Autodesk Inventor part; units mm, degrees
(part 3 of 5)
sketch "Sketch8" plane through (0, 0, 3) normal (0, 0, 1) x (1, 0, 0)
  line L0 (80.4, 215) -> (-78, 215) projected
  line L1 (-78, 215) -> (-78, 46.0635) projected
  line L2 (-78, 46.0635) -> (-75, 46.0635) projected
  line L3 (-75, 46.0635) -> (-75, 40.8932) projected
  line L4 (-75, 40.8932) -> (-78, 40.8932) projected
  line L5 (-78, 40.8932) -> (-78, 30.6062) projected
  line L6 (-78, 30.6062) -> (-75, 30.6062) projected
  line L7 (-75, 30.6062) -> (-75, 20.5478) projected
  line L8 (-75, 20.5478) -> (-78, 20.5478) projected
  line L9 (-78, 20.5478) -> (-78, 10.2608) projected
  line L10 (-78, 10.2608) -> (-75, 10.2608) projected
  line L11 (-75, 10.2608) -> (-75, -0.1068) projected
  line L12 (-75, -0.1068) -> (-78, -0.1068) projected
  line L13 (-78, -0.1068) -> (-78, -10.3938) projected
  line L14 (-78, -10.3938) -> (-75, -10.3938) projected
  line L15 (-75, -10.3938) -> (-75, -20.4522) projected
  line L16 (-75, -20.4522) -> (-78, -20.4522) projected
  line L17 (-78, -20.4522) -> (-78, -30.7392) projected
  line L18 (-78, -30.7392) -> (-75, -30.7392) projected
  line L19 (-75, -30.7392) -> (-75, -41.1068) projected
  line L20 (-75, -41.1068) -> (-78, -41.1068) projected
  line L21 (-78, -41.1068) -> (-78, -51.3938) projected
  line L22 (-78, -51.3938) -> (-75, -51.3938) projected
  line L23 (-75, -51.3938) -> (-75, -61.4522) projected
  line L24 (-75, -61.4522) -> (-78, -61.4522) projected
  line L25 (-78, -61.4522) -> (-78, -71.7392) projected
  line L26 (-78, -71.7392) -> (-75, -71.7392) projected
  line L27 (-75, -71.7392) -> (-75, -82.1068) projected
  line L28 (-75, -82.1068) -> (-78, -82.1068) projected
  line L29 (-78, -82.1068) -> (-78, -92.3938) projected
  line L30 (-78, -92.3938) -> (-75, -92.3938) projected
  line L31 (-75, -92.3938) -> (-75, -102.4522) projected
  line L32 (-75, -102.4522) -> (-78, -102.4522) projected
  line L33 (-78, -102.4522) -> (-78, -112.7392) projected
  line L34 (-78, -112.7392) -> (-75, -112.7392) projected
  line L35 (-75, -112.7392) -> (-75, -130) projected
  line L36 (-75, -130) -> (-25.3933, -130) projected
  line L37 (-25.3933, -130) -> (-25.3933, -147.5) projected
  line L38 (-25.3933, -147.5) -> (23.6067, -147.5) projected
  line L39 (23.6067, -147.5) -> (23.6067, -130) projected
  line L40 (23.6067, -130) -> (98, -130) projected
  line L41 (98, -130) -> (98, 184.5) projected
  line L42 (98, 184.5) -> (80.4, 184.5) projected
  line L43 (80.4, 184.5) -> (80.4, 215) projected
  circle A0 centre (88, 174.5) radius 2.25 projected
  circle A1 centre (88, 131.8987) radius 2.25 projected
  circle A2 centre (88, 58.3987) radius 2.25 projected
  circle A3 centre (88, -117.6237) radius 2.25 projected
  circle A4 centre (-19.3694, 126.1487) radius 1.2 projected
  circle A5 centre (52.1306, 126.1487) radius 1.2 projected
  circle A6 centre (52.1306, 137.6487) radius 1.2 projected
  circle A7 centre (52.1306, 209.1487) radius 1.2 projected
  circle A8 centre (52.1306, 54.6487) radius 1.2 projected
  circle A9 centre (-19.3694, 137.6487) radius 1.2 projected
  circle A10 centre (-19.3694, 209.1487) radius 1.2 projected
  circle A11 centre (-19.3694, 54.6487) radius 1.2 projected
  circle A12 centre (-17.8933, -140) radius 2.25 projected
  circle A13 centre (16.1067, -140) radius 2.25 projected
  line L44 (-58.9404, 10.4643) -> (-58.9404, 20.3443) projected
  arc A14 (-55.9404, 23.3443) -> (-58.9404, 20.3443) centre (-55.9404, 20.3443) ccw projected
  line L45 (-55.9404, 23.3443) -> (31.7396, 23.3443) projected
  arc A15 (34.7396, 20.3443) -> (31.7396, 23.3443) centre (31.7396, 20.3443) ccw projected
  line L46 (34.7396, 20.3443) -> (34.7396, 10.4643) projected
  arc A16 (31.7396, 7.4643) -> (34.7396, 10.4643) centre (31.7396, 10.4643) ccw projected
  line L47 (31.7396, 7.4643) -> (-55.9404, 7.4643) projected
  arc A17 (-58.9404, 10.4643) -> (-55.9404, 7.4643) centre (-55.9404, 10.4643) ccw projected
  line L48 (-58.9404, 30.8097) -> (-58.9404, 40.6897) projected
  arc A18 (-55.9404, 43.6897) -> (-58.9404, 40.6897) centre (-55.9404, 40.6897) ccw projected
  line L49 (-55.9404, 43.6897) -> (31.7396, 43.6897) projected
  arc A19 (34.7396, 40.6897) -> (31.7396, 43.6897) centre (31.7396, 40.6897) ccw projected
  line L50 (34.7396, 40.6897) -> (34.7396, 30.8097) projected
  arc A20 (31.7396, 27.8097) -> (34.7396, 30.8097) centre (31.7396, 30.8097) ccw projected
  line L51 (31.7396, 27.8097) -> (-55.9404, 27.8097) projected
  arc A21 (-58.9404, 30.8097) -> (-55.9404, 27.8097) centre (-55.9404, 30.8097) ccw projected
  arc A22 (-55.9404, 2.9989) -> (-58.9404, -0.0011) centre (-55.9404, -0.0011) ccw projected
  line L52 (-55.9404, 2.9989) -> (31.7396, 2.9989) projected
  arc A23 (34.7396, -0.0011) -> (31.7396, 2.9989) centre (31.7396, -0.0011) ccw projected
  line L53 (34.7396, -0.0011) -> (34.7396, -9.8811) projected
  arc A24 (31.7396, -12.8811) -> (34.7396, -9.8811) centre (31.7396, -9.8811) ccw projected
  line L54 (31.7396, -12.8811) -> (-55.9404, -12.8811) projected
  arc A25 (-58.9404, -9.8811) -> (-55.9404, -12.8811) centre (-55.9404, -9.8811) ccw projected
  line L55 (-58.9404, -9.8811) -> (-58.9404, -0.0011) projected
  arc A26 (-55.9404, -37.6919) -> (-58.9404, -40.6919) centre (-55.9404, -40.6919) ccw projected
  line L56 (-55.9404, -37.6919) -> (31.7396, -37.6919) projected
  arc A27 (34.7396, -40.6919) -> (31.7396, -37.6919) centre (31.7396, -40.6919) ccw projected
  line L57 (34.7396, -40.6919) -> (34.7396, -50.5719) projected
  arc A28 (31.7396, -53.5719) -> (34.7396, -50.5719) centre (31.7396, -50.5719) ccw projected
  line L58 (31.7396, -53.5719) -> (-55.9404, -53.5719) projected
  arc A29 (-58.9404, -50.5719) -> (-55.9404, -53.5719) centre (-55.9404, -50.5719) ccw projected
  line L59 (-58.9404, -50.5719) -> (-58.9404, -40.6919) projected
  line L60 (-55.9404, -58.0373) -> (31.7396, -58.0373) projected
  arc A30 (34.7396, -61.0373) -> (31.7396, -58.0373) centre (31.7396, -61.0373) ccw projected
  line L61 (34.7396, -61.0373) -> (34.7396, -70.9173) projected
  arc A31 (31.7396, -73.9173) -> (34.7396, -70.9173) centre (31.7396, -70.9173) ccw projected
  line L62 (31.7396, -73.9173) -> (-55.9404, -73.9173) projected
  arc A32 (-58.9404, -70.9173) -> (-55.9404, -73.9173) centre (-55.9404, -70.9173) ccw projected
  line L63 (-58.9404, -70.9173) -> (-58.9404, -61.0373) projected
  arc A33 (-55.9404, -58.0373) -> (-58.9404, -61.0373) centre (-55.9404, -61.0373) ccw projected
  line L64 (31.7396, -33.2265) -> (-55.9404, -33.2265) projected
  arc A34 (-58.9404, -30.2265) -> (-55.9404, -33.2265) centre (-55.9404, -30.2265) ccw projected
  line L65 (-58.9404, -30.2265) -> (-58.9404, -20.3465) projected
  arc A35 (-55.9404, -17.3465) -> (-58.9404, -20.3465) centre (-55.9404, -20.3465) ccw projected
  line L66 (-55.9404, -17.3465) -> (31.7396, -17.3465) projected
  arc A36 (34.7396, -20.3465) -> (31.7396, -17.3465) centre (31.7396, -20.3465) ccw projected
  line L67 (34.7396, -20.3465) -> (34.7396, -30.2265) projected
  arc A37 (31.7396, -33.2265) -> (34.7396, -30.2265) centre (31.7396, -30.2265) ccw projected
  arc A38 (34.7396, -81.3827) -> (31.7396, -78.3827) centre (31.7396, -81.3827) ccw projected
  line L68 (34.7396, -81.3827) -> (34.7396, -91.2627) projected
  arc A39 (31.7396, -94.2627) -> (34.7396, -91.2627) centre (31.7396, -91.2627) ccw projected
  line L69 (31.7396, -94.2627) -> (-55.9404, -94.2627) projected
  arc A40 (-58.9404, -91.2627) -> (-55.9404, -94.2627) centre (-55.9404, -91.2627) ccw projected
  line L70 (-58.9404, -91.2627) -> (-58.9404, -81.3827) projected
  arc A41 (-55.9404, -78.3827) -> (-58.9404, -81.3827) centre (-55.9404, -81.3827) ccw projected
  line L71 (-55.9404, -78.3827) -> (31.7396, -78.3827) projected
  arc A42 (31.7396, -114.6081) -> (34.7396, -111.6081) centre (31.7396, -111.6081) ccw projected
  line L72 (31.7396, -114.6081) -> (-55.9404, -114.6081) projected
  arc A43 (-58.9404, -111.6081) -> (-55.9404, -114.6081) centre (-55.9404, -111.6081) ccw projected
  line L73 (-58.9404, -111.6081) -> (-58.9404, -101.7281) projected
  arc A44 (-55.9404, -98.7281) -> (-58.9404, -101.7281) centre (-55.9404, -101.7281) ccw projected
  line L74 (-55.9404, -98.7281) -> (31.7396, -98.7281) projected
  arc A45 (34.7396, -101.7281) -> (31.7396, -98.7281) centre (31.7396, -101.7281) ccw projected
  line L75 (34.7396, -101.7281) -> (34.7396, -111.6081) projected
  arc A46 (-6.9692, 54.8876) -> (4.019, 51.5987) centre (4.019, 71.5987) ccw projected
  arc A47 (-13.8416, 60.5179) -> (-6.9692, 54.8876) centre (16.3806, 90.3987) ccw projected
  arc A48 (-19.6194, 74.5794) -> (-13.8416, 60.5179) centre (0.3806, 74.5794) ccw projected
  line L76 (-19.6194, 74.5794) -> (-19.6194, 106.218) projected
  arc A49 (-13.8416, 120.2796) -> (-19.6194, 106.218) centre (0.3806, 106.218) ccw projected
  arc A50 (-6.9692, 125.9099) -> (-13.8416, 120.2796) centre (16.3806, 90.3987) ccw projected
  arc A51 (4.019, 129.1987) -> (-6.9692, 125.9099) centre (4.019, 109.1987) ccw projected
  line L77 (4.019, 129.1987) -> (28.7422, 129.1987) projected
  arc A52 (39.7304, 125.9099) -> (28.7422, 129.1987) centre (28.7422, 109.1987) ccw projected
  arc A53 (46.6028, 120.2796) -> (39.7304, 125.9099) centre (16.3806, 90.3987) ccw projected
  arc A54 (52.3806, 106.218) -> (46.6028, 120.2796) centre (32.3806, 106.218) ccw projected
  line L78 (52.3806, 106.218) -> (52.3806, 74.5794) projected
  arc A55 (46.6028, 60.5179) -> (52.3806, 74.5794) centre (32.3806, 74.5794) ccw projected
  arc A56 (39.7304, 54.8876) -> (46.6028, 60.5179) centre (16.3806, 90.3987) ccw projected
  arc A57 (28.7422, 51.5987) -> (39.7304, 54.8876) centre (28.7422, 71.5987) ccw projected
  line L79 (28.7422, 51.5987) -> (4.019, 51.5987) projected
  arc A58 (-6.9692, 137.8876) -> (4.019, 134.5987) centre (4.019, 154.5987) ccw projected
  arc A59 (-13.8416, 143.5179) -> (-6.9692, 137.8876) centre (16.3806, 173.3987) ccw projected
  arc A60 (-19.6194, 157.5794) -> (-13.8416, 143.5179) centre (0.3806, 157.5794) ccw projected
  line L80 (-19.6194, 157.5794) -> (-19.6194, 189.218) projected
  arc A61 (-13.8416, 203.2796) -> (-19.6194, 189.218) centre (0.3806, 189.218) ccw projected
  arc A62 (-6.9692, 208.9099) -> (-13.8416, 203.2796) centre (16.3806, 173.3987) ccw projected
  arc A63 (4.019, 212.1987) -> (-6.9692, 208.9099) centre (4.019, 192.1987) ccw projected
  line L81 (4.019, 212.1987) -> (28.7422, 212.1987) projected
  arc A64 (39.7304, 208.9099) -> (28.7422, 212.1987) centre (28.7422, 192.1987) ccw projected
  arc A65 (46.6028, 203.2796) -> (39.7304, 208.9099) centre (16.3806, 173.3987) ccw projected
  arc A66 (52.3806, 189.218) -> (46.6028, 203.2796) centre (32.3806, 189.218) ccw projected
  line L82 (52.3806, 189.218) -> (52.3806, 157.5794) projected
  arc A67 (46.6028, 143.5179) -> (52.3806, 157.5794) centre (32.3806, 157.5794) ccw projected
  arc A68 (39.7304, 137.8876) -> (46.6028, 143.5179) centre (16.3806, 173.3987) ccw projected
  arc A69 (28.7422, 134.5987) -> (39.7304, 137.8876) centre (28.7422, 154.5987) ccw projected
  line L83 (28.7422, 134.5987) -> (4.019, 134.5987) projected
  line L84 (-69.3194, 50.0635) -> (-69.3194, 207.0635) projected
  arc A70 (-68.3194, 208.0635) -> (-69.3194, 207.0635) centre (-68.3194, 207.0635) ccw projected
  line L85 (-68.3194, 208.0635) -> (-25.6194, 208.0635) projected
  arc A71 (-24.6194, 207.0635) -> (-25.6194, 208.0635) centre (-25.6194, 207.0635) ccw projected
  line L86 (-24.6194, 207.0635) -> (-24.6194, 50.0635) projected
  arc A72 (-25.6194, 49.0635) -> (-24.6194, 50.0635) centre (-25.6194, 50.0635) ccw projected
  line L87 (-25.6194, 49.0635) -> (-68.3194, 49.0635) projected
  arc A73 (-69.3194, 50.0635) -> (-68.3194, 49.0635) centre (-68.3194, 50.0635) ccw projected
  line L88 (64, 48.3987) -> (64, -109.7094) projected
  arc A74 (63.7071, -110.4166) -> (64, -109.7094) centre (63, -109.7094) ccw projected
  line L89 (63.7071, -110.4166) -> (59.2929, -114.8308) projected
  arc A75 (58.5858, -115.1237) -> (59.2929, -114.8308) centre (58.5858, -114.1237) ccw projected
  line L90 (58.5858, -115.1237) -> (43.2196, -115.1237) projected
  arc A76 (42.2196, -114.1237) -> (43.2196, -115.1237) centre (43.2196, -114.1237) ccw projected
  line L91 (42.2196, -114.1237) -> (42.2196, -104.6674) projected
  arc A77 (42.2196, -104.6674) -> (40.773, -102.7455) centre (40.2196, -104.6674) ccw projected
  arc A78 (39.7673, -102.1811) -> (40.773, -102.7455) centre (41.4696, -100.3262) ccw projected
  arc A79 (39.1196, -100.7076) -> (39.7673, -102.1811) centre (41.1196, -100.7076) ccw projected
  line L92 (39.1196, -100.7076) -> (39.1196, -95.7515) projected
  arc A80 (39.7673, -94.2779) -> (39.1196, -95.7515) centre (41.1196, -95.7515) ccw projected
  arc A81 (39.937, -94.1354) -> (39.7673, -94.2779) centre (41.4696, -96.1328) ccw projected
  arc A82 (39.937, -94.1354) -> (40.7196, -92.5486) centre (38.7196, -92.5486) ccw projected
  line L93 (40.7196, -92.5486) -> (40.7196, -83.4104) projected
  arc A83 (40.7196, -83.4104) -> (39.937, -81.8236) centre (38.7196, -83.4104) ccw projected
  arc A84 (39.7673, -81.6811) -> (39.937, -81.8236) centre (41.4696, -79.8262) ccw projected
  arc A85 (39.1196, -80.2076) -> (39.7673, -81.6811) centre (41.1196, -80.2076) ccw projected
  line L94 (39.1196, -80.2076) -> (39.1196, -75.2515) projected
  arc A86 (39.7673, -73.7779) -> (39.1196, -75.2515) centre (41.1196, -75.2515) ccw projected
  arc A87 (39.937, -73.6354) -> (39.7673, -73.7779) centre (41.4696, -75.6328) ccw projected
  arc A88 (39.937, -73.6354) -> (40.7196, -72.0486) centre (38.7196, -72.0486) ccw projected
  line L95 (40.7196, -72.0486) -> (40.7196, -62.9104) projected
  arc A89 (40.7196, -62.9104) -> (39.937, -61.3236) centre (38.7196, -62.9104) ccw projected
  arc A90 (39.7673, -61.1811) -> (39.937, -61.3236) centre (41.4696, -59.3262) ccw projected
  arc A91 (39.1196, -59.7076) -> (39.7673, -61.1811) centre (41.1196, -59.7076) ccw projected
  line L96 (39.1196, -59.7076) -> (39.1196, -54.7515) projected
  arc A92 (39.7673, -53.2779) -> (39.1196, -54.7515) centre (41.1196, -54.7515) ccw projected
  arc A93 (39.937, -53.1354) -> (39.7673, -53.2779) centre (41.4696, -55.1328) ccw projected
  arc A94 (39.937, -53.1354) -> (40.7196, -51.5486) centre (38.7196, -51.5486) ccw projected
  line L97 (40.7196, -51.5486) -> (40.7196, -42.4104) projected
  arc A95 (40.7196, -42.4104) -> (39.937, -40.8236) centre (38.7196, -42.4104) ccw projected
  arc A96 (39.7673, -40.6811) -> (39.937, -40.8236) centre (41.4696, -38.8262) ccw projected
  arc A97 (39.1196, -39.2076) -> (39.7673, -40.6811) centre (41.1196, -39.2076) ccw projected
  line L98 (39.1196, -39.2076) -> (39.1196, -34.2515) projected
  arc A98 (39.7673, -32.7779) -> (39.1196, -34.2515) centre (41.1196, -34.2515) ccw projected
  arc A99 (39.937, -32.6354) -> (39.7673, -32.7779) centre (41.4696, -34.6328) ccw projected
  arc A100 (39.937, -32.6354) -> (40.7196, -31.0486) centre (38.7196, -31.0486) ccw projected
  line L99 (40.7196, -31.0486) -> (40.7196, -21.9104) projected
  arc A101 (40.7196, -21.9104) -> (39.937, -20.3236) centre (38.7196, -21.9104) ccw projected
  arc A102 (39.7673, -20.1811) -> (39.937, -20.3236) centre (41.4696, -18.3262) ccw projected
  arc A103 (39.1196, -18.7076) -> (39.7673, -20.1811) centre (41.1196, -18.7076) ccw projected
  line L100 (39.1196, -18.7076) -> (39.1196, -13.7515) projected
  arc A104 (39.7673, -12.2779) -> (39.1196, -13.7515) centre (41.1196, -13.7515) ccw projected
  arc A105 (39.937, -12.1354) -> (39.7673, -12.2779) centre (41.4696, -14.1328) ccw projected
  arc A106 (39.937, -12.1354) -> (40.7196, -10.5486) centre (38.7196, -10.5486) ccw projected
  line L101 (40.7196, -10.5486) -> (40.7196, -1.4104) projected
  arc A107 (40.7196, -1.4104) -> (39.937, 0.1764) centre (38.7196, -1.4104) ccw projected
  arc A108 (39.7673, 0.3189) -> (39.937, 0.1764) centre (41.4696, 2.1738) ccw projected
  arc A109 (39.1196, 1.7924) -> (39.7673, 0.3189) centre (41.1196, 1.7924) ccw projected
  line L102 (39.1196, 1.7924) -> (39.1196, 6.7485) projected
  arc A110 (39.7673, 8.2221) -> (39.1196, 6.7485) centre (41.1196, 6.7485) ccw projected
  arc A111 (39.937, 8.3646) -> (39.7673, 8.2221) centre (41.4696, 6.3672) ccw projected
  arc A112 (39.937, 8.3646) -> (40.7196, 9.9514) centre (38.7196, 9.9514) ccw projected
  line L103 (40.7196, 9.9514) -> (40.7196, 19.0896) projected
  arc A113 (40.7196, 19.0896) -> (39.937, 20.6764) centre (38.7196, 19.0896) ccw projected
  arc A114 (39.7673, 20.8189) -> (39.937, 20.6764) centre (41.4696, 22.6738) ccw projected
  arc A115 (39.1196, 22.2924) -> (39.7673, 20.8189) centre (41.1196, 22.2924) ccw projected
  line L104 (39.1196, 22.2924) -> (39.1196, 27.2485) projected
  arc A116 (39.7673, 28.7221) -> (39.1196, 27.2485) centre (41.1196, 27.2485) ccw projected
  arc A117 (39.937, 28.8646) -> (39.7673, 28.7221) centre (41.4696, 26.8672) ccw projected
  arc A118 (39.937, 28.8646) -> (40.7196, 30.4514) centre (38.7196, 30.4514) ccw projected
  line L105 (40.7196, 30.4514) -> (40.7196, 39.5896) projected
  arc A119 (40.7196, 39.5896) -> (39.937, 41.1764) centre (38.7196, 39.5896) ccw projected
  arc A120 (39.7673, 41.3189) -> (39.937, 41.1764) centre (41.4696, 43.1738) ccw projected
  arc A121 (39.1196, 42.7924) -> (39.7673, 41.3189) centre (41.1196, 42.7924) ccw projected
  line L106 (39.1196, 42.7924) -> (39.1196, 47.7485) projected
  arc A122 (39.7673, 49.2221) -> (39.1196, 47.7485) centre (41.1196, 47.7485) ccw projected
  arc A123 (43.3362, 49.0566) -> (39.7673, 49.2221) centre (41.4696, 47.3672) ccw projected
  arc A124 (43.3362, 49.0566) -> (44.819, 48.3987) centre (44.819, 50.3987) ccw projected
  line L107 (44.819, 48.3987) -> (64, 48.3987) projected
  point P0 (0, 0)
extrude "Extrusion9" add sketch "Sketch8" against normal up to surface (3 mm away) contours A4 | A5 | A6 | A7 | A8 | A9 | A10 | A11 | A47 A48 L76 A49 A50 A51 L77 A52 A53 A54 L78 A55 A56 A57 L79 A46 | A59 A60 L80 A61 A62 A63 L81 A64 A65 A66 L82 A67 A68 A69 L83 A58
sketch "Sketch9" plane through (0, 0, 3) normal (0, 0, 1) x (1, 0, 0)
  circle A0 centre (-12.181, 125.9009) radius 1.2
  circle A1 centre (59.319, 125.9009) radius 1.2
  circle A2 centre (59.319, 137.4009) radius 1.2
  circle A3 centre (59.319, 208.9009) radius 1.2
  circle A4 centre (59.319, 54.4009) radius 1.2
  circle A5 centre (-12.181, 137.4009) radius 1.2
  circle A6 centre (-12.181, 208.9009) radius 1.2
  circle A7 centre (-12.181, 54.4009) radius 1.2
  arc A8 (0.2192, 54.6398) -> (11.2074, 51.3509) centre (11.2074, 71.3509) ccw
  arc A9 (-6.6532, 60.27) -> (0.2192, 54.6398) centre (23.569, 90.1509) ccw
  arc A10 (-12.431, 74.3316) -> (-6.6532, 60.27) centre (7.569, 74.3316) ccw
  line L0 (-12.431, 74.3316) -> (-12.431, 105.9702)
  arc A11 (-6.6532, 120.0317) -> (-12.431, 105.9702) centre (7.569, 105.9702) ccw
  arc A12 (0.2192, 125.662) -> (-6.6532, 120.0317) centre (23.569, 90.1509) ccw
  arc A13 (11.2074, 128.9509) -> (0.2192, 125.662) centre (11.2074, 108.9509) ccw
  line L1 (11.2074, 128.9509) -> (35.9306, 128.9509)
  arc A14 (46.9188, 125.662) -> (35.9306, 128.9509) centre (35.9306, 108.9509) ccw
  arc A15 (53.7912, 120.0317) -> (46.9188, 125.662) centre (23.569, 90.1509) ccw
  arc A16 (59.569, 105.9702) -> (53.7912, 120.0317) centre (39.569, 105.9702) ccw
  line L2 (59.569, 105.9702) -> (59.569, 74.3316)
  arc A17 (53.7912, 60.27) -> (59.569, 74.3316) centre (39.569, 74.3316) ccw
  arc A18 (46.9188, 54.6398) -> (53.7912, 60.27) centre (23.569, 90.1509) ccw
  arc A19 (35.9306, 51.3509) -> (46.9188, 54.6398) centre (35.9306, 71.3509) ccw
  line L3 (35.9306, 51.3509) -> (11.2074, 51.3509)
  arc A20 (0.2192, 137.6398) -> (11.2074, 134.3509) centre (11.2074, 154.3509) ccw
  arc A21 (-6.6532, 143.27) -> (0.2192, 137.6398) centre (23.569, 173.1509) ccw
  arc A22 (-12.431, 157.3316) -> (-6.6532, 143.27) centre (7.569, 157.3316) ccw
  line L4 (-12.431, 157.3316) -> (-12.431, 188.9702)
  arc A23 (-6.6532, 203.0317) -> (-12.431, 188.9702) centre (7.569, 188.9702) ccw
  arc A24 (0.2192, 208.662) -> (-6.6532, 203.0317) centre (23.569, 173.1509) ccw
  arc A25 (11.2074, 211.9509) -> (0.2192, 208.662) centre (11.2074, 191.9509) ccw
  line L5 (11.2074, 211.9509) -> (35.9306, 211.9509)
  arc A26 (46.9188, 208.662) -> (35.9306, 211.9509) centre (35.9306, 191.9509) ccw
  arc A27 (53.7912, 203.0317) -> (46.9188, 208.662) centre (23.569, 173.1509) ccw
  arc A28 (59.569, 188.9702) -> (53.7912, 203.0317) centre (39.569, 188.9702) ccw
  line L6 (59.569, 188.9702) -> (59.569, 157.3316)
  arc A29 (53.7912, 143.27) -> (59.569, 157.3316) centre (39.569, 157.3316) ccw
  arc A30 (46.9188, 137.6398) -> (53.7912, 143.27) centre (23.569, 173.1509) ccw
  arc A31 (35.9306, 134.3509) -> (46.9188, 137.6398) centre (35.9306, 154.3509) ccw
  line L7 (35.9306, 134.3509) -> (11.2074, 134.3509)
  point P0 (0, 0)
  constraints: 48 point on circle, 32 centre point, 16 end point
extrude "Extrusion10" cut sketch "Sketch9" against normal blind 10
sketch "Sketch10" plane through (0, 0, 3) normal (0, 0, 1) x (1, 0, 0)
  arc A0 (46.9188, 54.6398) -> (53.7912, 60.27) centre (23.569, 90.1509) ccw projected
  arc A1 (35.9306, 51.3509) -> (46.9188, 54.6398) centre (35.9306, 71.3509) ccw projected
  line L0 (35.9306, 51.3509) -> (11.2074, 51.3509) projected
  arc A2 (0.2192, 54.6398) -> (11.2074, 51.3509) centre (11.2074, 71.3509) ccw projected
  arc A3 (-6.6532, 60.27) -> (0.2192, 54.6398) centre (23.569, 90.1509) ccw projected
  arc A4 (-12.431, 74.3316) -> (-6.6532, 60.27) centre (7.569, 74.3316) ccw projected
  line L1 (-12.431, 74.3316) -> (-12.431, 105.9702) projected
  arc A5 (-6.6532, 120.0317) -> (-12.431, 105.9702) centre (7.569, 105.9702) ccw projected
  arc A6 (0.2192, 125.662) -> (-6.6532, 120.0317) centre (23.569, 90.1509) ccw projected
  arc A7 (11.2074, 128.9509) -> (0.2192, 125.662) centre (11.2074, 108.9509) ccw projected
  line L2 (11.2074, 128.9509) -> (35.9306, 128.9509) projected
  arc A8 (46.9188, 125.662) -> (35.9306, 128.9509) centre (35.9306, 108.9509) ccw projected
  arc A9 (53.7912, 120.0317) -> (46.9188, 125.662) centre (23.569, 90.1509) ccw projected
  arc A10 (59.569, 105.9702) -> (53.7912, 120.0317) centre (39.569, 105.9702) ccw projected
  line L3 (59.569, 105.9702) -> (59.569, 74.3316) projected
  arc A11 (53.7912, 60.27) -> (59.569, 74.3316) centre (39.569, 74.3316) ccw projected
  circle A12 centre (-12.181, 208.9009) radius 1.2 projected
  circle A13 centre (59.319, 137.4009) radius 1.2 projected
  circle A14 centre (-12.181, 137.4009) radius 1.2 projected
  circle A15 centre (59.319, 54.4009) radius 1.2 projected
  circle A16 centre (-12.181, 125.9009) radius 1.2 projected
  circle A17 centre (59.319, 125.9009) radius 1.2 projected
  circle A18 centre (59.319, 208.9009) radius 1.2 projected
  circle A19 centre (-12.181, 54.4009) radius 1.2 projected
  arc A20 (46.9188, 137.6398) -> (53.7912, 143.27) centre (23.569, 173.1509) ccw projected
  arc A21 (35.9306, 134.3509) -> (46.9188, 137.6398) centre (35.9306, 154.3509) ccw projected
  line L4 (35.9306, 134.3509) -> (11.2074, 134.3509) projected
  arc A22 (0.2192, 137.6398) -> (11.2074, 134.3509) centre (11.2074, 154.3509) ccw projected
  arc A23 (-6.6532, 143.27) -> (0.2192, 137.6398) centre (23.569, 173.1509) ccw projected
  arc A24 (-12.431, 157.3316) -> (-6.6532, 143.27) centre (7.569, 157.3316) ccw projected
  line L5 (-12.431, 157.3316) -> (-12.431, 188.9702) projected
  arc A25 (-6.6532, 203.0317) -> (-12.431, 188.9702) centre (7.569, 188.9702) ccw projected
  arc A26 (0.2192, 208.662) -> (-6.6532, 203.0317) centre (23.569, 173.1509) ccw projected
  arc A27 (11.2074, 211.9509) -> (0.2192, 208.662) centre (11.2074, 191.9509) ccw projected
  line L6 (11.2074, 211.9509) -> (35.9306, 211.9509) projected
  arc A28 (46.9188, 208.662) -> (35.9306, 211.9509) centre (35.9306, 191.9509) ccw projected
  arc A29 (53.7912, 203.0317) -> (46.9188, 208.662) centre (23.569, 173.1509) ccw projected
  arc A30 (59.569, 188.9702) -> (53.7912, 203.0317) centre (39.569, 188.9702) ccw projected
  line L7 (59.569, 188.9702) -> (59.569, 157.3316) projected
  arc A31 (53.7912, 143.27) -> (59.569, 157.3316) centre (39.569, 157.3316) ccw projected
  line L8 (80.4, 215) -> (-78, 215) projected
  line L9 (-78, 215) -> (-78, 46.0635) projected
  line L10 (-78, 46.0635) -> (-75, 46.0635) projected
  line L11 (-75, 46.0635) -> (-75, 40.8932) projected
  line L12 (-75, 40.8932) -> (-78, 40.8932) projected
  line L13 (-78, 40.8932) -> (-78, 30.6062) projected
  line L14 (-78, 30.6062) -> (-75, 30.6062) projected
  line L15 (-75, 30.6062) -> (-75, 20.5478) projected
  line L16 (-75, 20.5478) -> (-78, 20.5478) projected
  line L17 (-78, 20.5478) -> (-78, 10.2608) projected
  line L18 (-78, 10.2608) -> (-75, 10.2608) projected
  line L19 (-75, 10.2608) -> (-75, -0.1068) projected
  line L20 (-75, -0.1068) -> (-78, -0.1068) projected
  line L21 (-78, -0.1068) -> (-78, -10.3938) projected
  line L22 (-78, -10.3938) -> (-75, -10.3938) projected
  line L23 (-75, -10.3938) -> (-75, -20.4522) projected
  line L24 (-75, -20.4522) -> (-78, -20.4522) projected
  line L25 (-78, -20.4522) -> (-78, -30.7392) projected
  line L26 (-78, -30.7392) -> (-75, -30.7392) projected
  line L27 (-75, -30.7392) -> (-75, -41.1068) projected
  line L28 (-75, -41.1068) -> (-78, -41.1068) projected
  line L29 (-78, -41.1068) -> (-78, -51.3938) projected
  line L30 (-78, -51.3938) -> (-75, -51.3938) projected
  line L31 (-75, -51.3938) -> (-75, -61.4522) projected
  line L32 (-75, -61.4522) -> (-78, -61.4522) projected
  line L33 (-78, -61.4522) -> (-78, -71.7392) projected
  line L34 (-78, -71.7392) -> (-75, -71.7392) projected
  line L35 (-75, -71.7392) -> (-75, -82.1068) projected
  line L36 (-75, -82.1068) -> (-78, -82.1068) projected
  line L37 (-78, -82.1068) -> (-78, -92.3938) projected
  line L38 (-78, -92.3938) -> (-75, -92.3938) projected
  line L39 (-75, -92.3938) -> (-75, -102.4522) projected
  line L40 (-75, -102.4522) -> (-78, -102.4522) projected
  line L41 (-78, -102.4522) -> (-78, -112.7392) projected
  line L42 (-78, -112.7392) -> (-75, -112.7392) projected
  line L43 (-75, -112.7392) -> (-75, -130) projected
  line L44 (-75, -130) -> (-25.3933, -130) projected
  line L45 (-25.3933, -130) -> (-25.3933, -147.5) projected
  line L46 (-25.3933, -147.5) -> (23.6067, -147.5) projected
  line L47 (23.6067, -147.5) -> (23.6067, -130) projected
  line L48 (23.6067, -130) -> (98, -130) projected
  line L49 (98, -130) -> (98, 184.5) projected
  line L50 (98, 184.5) -> (80.4, 184.5) projected
  line L51 (80.4, 184.5) -> (80.4, 215) projected
  circle A32 centre (88, 174.5) radius 2.25 projected
  circle A33 centre (88, 131.8987) radius 2.25 projected
  circle A34 centre (88, 58.3987) radius 2.25 projected
  circle A35 centre (88, -117.6237) radius 2.25 projected
  circle A36 centre (-17.8933, -140) radius 2.25 projected
  circle A37 centre (16.1067, -140) radius 2.25 projected
  line L52 (-58.9404, 10.4643) -> (-58.9404, 20.3443) projected
  arc A38 (-55.9404, 23.3443) -> (-58.9404, 20.3443) centre (-55.9404, 20.3443) ccw projected
  line L53 (-55.9404, 23.3443) -> (31.7396, 23.3443) projected
  arc A39 (34.7396, 20.3443) -> (31.7396, 23.3443) centre (31.7396, 20.3443) ccw projected
  line L54 (34.7396, 20.3443) -> (34.7396, 10.4643) projected
  arc A40 (31.7396, 7.4643) -> (34.7396, 10.4643) centre (31.7396, 10.4643) ccw projected
  line L55 (31.7396, 7.4643) -> (-55.9404, 7.4643) projected
  arc A41 (-58.9404, 10.4643) -> (-55.9404, 7.4643) centre (-55.9404, 10.4643) ccw projected
  line L56 (-58.9404, 30.8097) -> (-58.9404, 40.6897) projected
  arc A42 (-55.9404, 43.6897) -> (-58.9404, 40.6897) centre (-55.9404, 40.6897) ccw projected
  line L57 (-55.9404, 43.6897) -> (31.7396, 43.6897) projected
  arc A43 (34.7396, 40.6897) -> (31.7396, 43.6897) centre (31.7396, 40.6897) ccw projected
  line L58 (34.7396, 40.6897) -> (34.7396, 30.8097) projected
  arc A44 (31.7396, 27.8097) -> (34.7396, 30.8097) centre (31.7396, 30.8097) ccw projected
  line L59 (31.7396, 27.8097) -> (-55.9404, 27.8097) projected
  arc A45 (-58.9404, 30.8097) -> (-55.9404, 27.8097) centre (-55.9404, 30.8097) ccw projected
  arc A46 (-55.9404, 2.9989) -> (-58.9404, -0.0011) centre (-55.9404, -0.0011) ccw projected
  line L60 (-55.9404, 2.9989) -> (31.7396, 2.9989) projected
  arc A47 (34.7396, -0.0011) -> (31.7396, 2.9989) centre (31.7396, -0.0011) ccw projected
  line L61 (34.7396, -0.0011) -> (34.7396, -9.8811) projected
  arc A48 (31.7396, -12.8811) -> (34.7396, -9.8811) centre (31.7396, -9.8811) ccw projected
  line L62 (31.7396, -12.8811) -> (-55.9404, -12.8811) projected
  arc A49 (-58.9404, -9.8811) -> (-55.9404, -12.8811) centre (-55.9404, -9.8811) ccw projected
  line L63 (-58.9404, -9.8811) -> (-58.9404, -0.0011) projected
  arc A50 (-55.9404, -37.6919) -> (-58.9404, -40.6919) centre (-55.9404, -40.6919) ccw projected
  line L64 (-55.9404, -37.6919) -> (31.7396, -37.6919) projected
  arc A51 (34.7396, -40.6919) -> (31.7396, -37.6919) centre (31.7396, -40.6919) ccw projected
  line L65 (34.7396, -40.6919) -> (34.7396, -50.5719) projected
  arc A52 (31.7396, -53.5719) -> (34.7396, -50.5719) centre (31.7396, -50.5719) ccw projected
  line L66 (31.7396, -53.5719) -> (-55.9404, -53.5719) projected
  arc A53 (-58.9404, -50.5719) -> (-55.9404, -53.5719) centre (-55.9404, -50.5719) ccw projected
  line L67 (-58.9404, -50.5719) -> (-58.9404, -40.6919) projected
  line L68 (-55.9404, -58.0373) -> (31.7396, -58.0373) projected
  arc A54 (34.7396, -61.0373) -> (31.7396, -58.0373) centre (31.7396, -61.0373) ccw projected
  line L69 (34.7396, -61.0373) -> (34.7396, -70.9173) projected
  arc A55 (31.7396, -73.9173) -> (34.7396, -70.9173) centre (31.7396, -70.9173) ccw projected
  line L70 (31.7396, -73.9173) -> (-55.9404, -73.9173) projected
  arc A56 (-58.9404, -70.9173) -> (-55.9404, -73.9173) centre (-55.9404, -70.9173) ccw projected
  line L71 (-58.9404, -70.9173) -> (-58.9404, -61.0373) projected
  arc A57 (-55.9404, -58.0373) -> (-58.9404, -61.0373) centre (-55.9404, -61.0373) ccw projected
  line L72 (31.7396, -33.2265) -> (-55.9404, -33.2265) projected
  arc A58 (-58.9404, -30.2265) -> (-55.9404, -33.2265) centre (-55.9404, -30.2265) ccw projected
  line L73 (-58.9404, -30.2265) -> (-58.9404, -20.3465) projected
  arc A59 (-55.9404, -17.3465) -> (-58.9404, -20.3465) centre (-55.9404, -20.3465) ccw projected
  line L74 (-55.9404, -17.3465) -> (31.7396, -17.3465) projected
  arc A60 (34.7396, -20.3465) -> (31.7396, -17.3465) centre (31.7396, -20.3465) ccw projected
  line L75 (34.7396, -20.3465) -> (34.7396, -30.2265) projected
  arc A61 (31.7396, -33.2265) -> (34.7396, -30.2265) centre (31.7396, -30.2265) ccw projected
  arc A62 (34.7396, -81.3827) -> (31.7396, -78.3827) centre (31.7396, -81.3827) ccw projected
  line L76 (34.7396, -81.3827) -> (34.7396, -91.2627) projected
  arc A63 (31.7396, -94.2627) -> (34.7396, -91.2627) centre (31.7396, -91.2627) ccw projected
  line L77 (31.7396, -94.2627) -> (-55.9404, -94.2627) projected
  arc A64 (-58.9404, -91.2627) -> (-55.9404, -94.2627) centre (-55.9404, -91.2627) ccw projected
  line L78 (-58.9404, -91.2627) -> (-58.9404, -81.3827) projected
  arc A65 (-55.9404, -78.3827) -> (-58.9404, -81.3827) centre (-55.9404, -81.3827) ccw projected
  line L79 (-55.9404, -78.3827) -> (31.7396, -78.3827) projected
  arc A66 (31.7396, -114.6081) -> (34.7396, -111.6081) centre (31.7396, -111.6081) ccw projected
  line L80 (31.7396, -114.6081) -> (-55.9404, -114.6081) projected
  arc A67 (-58.9404, -111.6081) -> (-55.9404, -114.6081) centre (-55.9404, -111.6081) ccw projected
  line L81 (-58.9404, -111.6081) -> (-58.9404, -101.7281) projected
  arc A68 (-55.9404, -98.7281) -> (-58.9404, -101.7281) centre (-55.9404, -101.7281) ccw projected
  line L82 (-55.9404, -98.7281) -> (31.7396, -98.7281) projected
  arc A69 (34.7396, -101.7281) -> (31.7396, -98.7281) centre (31.7396, -101.7281) ccw projected
  line L83 (34.7396, -101.7281) -> (34.7396, -111.6081) projected
  line L84 (-69.3194, 50.0635) -> (-69.3194, 207.0635) projected
  arc A70 (-68.3194, 208.0635) -> (-69.3194, 207.0635) centre (-68.3194, 207.0635) ccw projected
  line L85 (-68.3194, 208.0635) -> (-25.6194, 208.0635) projected
  arc A71 (-24.6194, 207.0635) -> (-25.6194, 208.0635) centre (-25.6194, 207.0635) ccw projected
  line L86 (-24.6194, 207.0635) -> (-24.6194, 50.0635) projected
  arc A72 (-25.6194, 49.0635) -> (-24.6194, 50.0635) centre (-25.6194, 50.0635) ccw projected
  line L87 (-25.6194, 49.0635) -> (-68.3194, 49.0635) projected
  arc A73 (-69.3194, 50.0635) -> (-68.3194, 49.0635) centre (-68.3194, 50.0635) ccw projected
  line L88 (64, 48.3987) -> (64, -109.7094) projected
  arc A74 (63.7071, -110.4166) -> (64, -109.7094) centre (63, -109.7094) ccw projected
  line L89 (63.7071, -110.4166) -> (59.2929, -114.8308) projected
  arc A75 (58.5858, -115.1237) -> (59.2929, -114.8308) centre (58.5858, -114.1237) ccw projected
  line L90 (58.5858, -115.1237) -> (43.2196, -115.1237) projected
  arc A76 (42.2196, -114.1237) -> (43.2196, -115.1237) centre (43.2196, -114.1237) ccw projected
  line L91 (42.2196, -114.1237) -> (42.2196, -104.6674) projected
  arc A77 (42.2196, -104.6674) -> (40.773, -102.7455) centre (40.2196, -104.6674) ccw projected
  arc A78 (39.7673, -102.1811) -> (40.773, -102.7455) centre (41.4696, -100.3262) ccw projected
  arc A79 (39.1196, -100.7076) -> (39.7673, -102.1811) centre (41.1196, -100.7076) ccw projected
  line L92 (39.1196, -100.7076) -> (39.1196, -95.7515) projected
  arc A80 (39.7673, -94.2779) -> (39.1196, -95.7515) centre (41.1196, -95.7515) ccw projected
  arc A81 (39.937, -94.1354) -> (39.7673, -94.2779) centre (41.4696, -96.1328) ccw projected
  arc A82 (39.937, -94.1354) -> (40.7196, -92.5486) centre (38.7196, -92.5486) ccw projected
  line L93 (40.7196, -92.5486) -> (40.7196, -83.4104) projected
  arc A83 (40.7196, -83.4104) -> (39.937, -81.8236) centre (38.7196, -83.4104) ccw projected
  arc A84 (39.7673, -81.6811) -> (39.937, -81.8236) centre (41.4696, -79.8262) ccw projected
  arc A85 (39.1196, -80.2076) -> (39.7673, -81.6811) centre (41.1196, -80.2076) ccw projected
  line L94 (39.1196, -80.2076) -> (39.1196, -75.2515) projected
  arc A86 (39.7673, -73.7779) -> (39.1196, -75.2515) centre (41.1196, -75.2515) ccw projected
  arc A87 (39.937, -73.6354) -> (39.7673, -73.7779) centre (41.4696, -75.6328) ccw projected
  arc A88 (39.937, -73.6354) -> (40.7196, -72.0486) centre (38.7196, -72.0486) ccw projected
  line L95 (40.7196, -72.0486) -> (40.7196, -62.9104) projected
  arc A89 (40.7196, -62.9104) -> (39.937, -61.3236) centre (38.7196, -62.9104) ccw projected
  arc A90 (39.7673, -61.1811) -> (39.937, -61.3236) centre (41.4696, -59.3262) ccw projected
  arc A91 (39.1196, -59.7076) -> (39.7673, -61.1811) centre (41.1196, -59.7076) ccw projected
  line L96 (39.1196, -59.7076) -> (39.1196, -54.7515) projected
  arc A92 (39.7673, -53.2779) -> (39.1196, -54.7515) centre (41.1196, -54.7515) ccw projected
  arc A93 (39.937, -53.1354) -> (39.7673, -53.2779) centre (41.4696, -55.1328) ccw projected
  arc A94 (39.937, -53.1354) -> (40.7196, -51.5486) centre (38.7196, -51.5486) ccw projected
  line L97 (40.7196, -51.5486) -> (40.7196, -42.4104) projected
  arc A95 (40.7196, -42.4104) -> (39.937, -40.8236) centre (38.7196, -42.4104) ccw projected
  arc A96 (39.7673, -40.6811) -> (39.937, -40.8236) centre (41.4696, -38.8262) ccw projected
  arc A97 (39.1196, -39.2076) -> (39.7673, -40.6811) centre (41.1196, -39.2076) ccw projected
  line L98 (39.1196, -39.2076) -> (39.1196, -34.2515) projected
  arc A98 (39.7673, -32.7779) -> (39.1196, -34.2515) centre (41.1196, -34.2515) ccw projected
  arc A99 (39.937, -32.6354) -> (39.7673, -32.7779) centre (41.4696, -34.6328) ccw projected
  arc A100 (39.937, -32.6354) -> (40.7196, -31.0486) centre (38.7196, -31.0486) ccw projected
  line L99 (40.7196, -31.0486) -> (40.7196, -21.9104) projected
  arc A101 (40.7196, -21.9104) -> (39.937, -20.3236) centre (38.7196, -21.9104) ccw projected
  arc A102 (39.7673, -20.1811) -> (39.937, -20.3236) centre (41.4696, -18.3262) ccw projected
  arc A103 (39.1196, -18.7076) -> (39.7673, -20.1811) centre (41.1196, -18.7076) ccw projected
  line L100 (39.1196, -18.7076) -> (39.1196, -13.7515) projected
  arc A104 (39.7673, -12.2779) -> (39.1196, -13.7515) centre (41.1196, -13.7515) ccw projected
  arc A105 (39.937, -12.1354) -> (39.7673, -12.2779) centre (41.4696, -14.1328) ccw projected
  arc A106 (39.937, -12.1354) -> (40.7196, -10.5486) centre (38.7196, -10.5486) ccw projected
  line L101 (40.7196, -10.5486) -> (40.7196, -1.4104) projected
  arc A107 (40.7196, -1.4104) -> (39.937, 0.1764) centre (38.7196, -1.4104) ccw projected
  arc A108 (39.7673, 0.3189) -> (39.937, 0.1764) centre (41.4696, 2.1738) ccw projected
  arc A109 (39.1196, 1.7924) -> (39.7673, 0.3189) centre (41.1196, 1.7924) ccw projected
  line L102 (39.1196, 1.7924) -> (39.1196, 6.7485) projected
  arc A110 (39.7673, 8.2221) -> (39.1196, 6.7485) centre (41.1196, 6.7485) ccw projected
  arc A111 (39.937, 8.3646) -> (39.7673, 8.2221) centre (41.4696, 6.3672) ccw projected
  arc A112 (39.937, 8.3646) -> (40.7196, 9.9514) centre (38.7196, 9.9514) ccw projected
  line L103 (40.7196, 9.9514) -> (40.7196, 19.0896) projected
  arc A113 (40.7196, 19.0896) -> (39.937, 20.6764) centre (38.7196, 19.0896) ccw projected
  arc A114 (39.7673, 20.8189) -> (39.937, 20.6764) centre (41.4696, 22.6738) ccw projected
  arc A115 (39.1196, 22.2924) -> (39.7673, 20.8189) centre (41.1196, 22.2924) ccw projected
  line L104 (39.1196, 22.2924) -> (39.1196, 27.2485) projected
  arc A116 (39.7673, 28.7221) -> (39.1196, 27.2485) centre (41.1196, 27.2485) ccw projected
  arc A117 (39.937, 28.8646) -> (39.7673, 28.7221) centre (41.4696, 26.8672) ccw projected
  arc A118 (39.937, 28.8646) -> (40.7196, 30.4514) centre (38.7196, 30.4514) ccw projected
  line L105 (40.7196, 30.4514) -> (40.7196, 39.5896) projected
  arc A119 (40.7196, 39.5896) -> (39.937, 41.1764) centre (38.7196, 39.5896) ccw projected
  arc A120 (39.7673, 41.3189) -> (39.937, 41.1764) centre (41.4696, 43.1738) ccw projected
  arc A121 (39.1196, 42.7924) -> (39.7673, 41.3189) centre (41.1196, 42.7924) ccw projected
  line L106 (39.1196, 42.7924) -> (39.1196, 47.7485) projected
  arc A122 (39.7673, 49.2221) -> (39.1196, 47.7485) centre (41.1196, 47.7485) ccw projected
  arc A123 (43.3362, 49.0566) -> (39.7673, 49.2221) centre (41.4696, 47.3672) ccw projected
  arc A124 (43.3362, 49.0566) -> (44.819, 48.3987) centre (44.819, 50.3987) ccw projected
  line L107 (44.819, 48.3987) -> (64, 48.3987) projected
  line L108 (-75, -129) -> (98, -129)
  line L109 (23.6067, -130) -> (23.6067, -129)
  line L110 (-75, -130) -> (-25.3933, -130) projected
  line L111 (-25.3933, -130) -> (-25.3933, -129)
  line L112 (-25.3933, -146.5) -> (23.6067, -146.5)
  line L113 (23.6067, -130) -> (23.6067, -147.5) projected
  point P0 (0, 0)
  dimension "d92" = 1
  dimension "d95" = 1
  constraints: 8 end point, 6 point on line, 3 perpendicular, 1 horizontal
  measures "d92" distance between parallel lines of L48 L108
  measures "d95" distance between parallel lines of L112 L46
extrude "Extrusion11" cut sketch "Sketch10" against normal blind 10 contours L49 L48 L109 L108 | L111 L44 L43 L108 | L47 L46 L45 L112
sketch "Sketch11" plane through (0, 0, 3) normal (0, 0, 1) x (1, 0, 0)
  circle A0 centre (-12.181, 137.4009) radius 1.2 projected
  arc A1 (0.2192, 137.6398) -> (11.2074, 134.3509) centre (11.2074, 154.3509) ccw projected
  line L0 (35.9306, 134.3509) -> (11.2074, 134.3509) projected
  arc A2 (35.9306, 134.3509) -> (46.9188, 137.6398) centre (35.9306, 154.3509) ccw projected
  arc A3 (46.9188, 137.6398) -> (53.7912, 143.27) centre (23.569, 173.1509) ccw projected
  arc A4 (53.7912, 143.27) -> (59.569, 157.3316) centre (39.569, 157.3316) ccw projected
  line L1 (59.569, 188.9702) -> (59.569, 157.3316) projected
  arc A5 (59.569, 188.9702) -> (53.7912, 203.0317) centre (39.569, 188.9702) ccw projected
  arc A6 (53.7912, 203.0317) -> (46.9188, 208.662) centre (23.569, 173.1509) ccw projected
  arc A7 (46.9188, 208.662) -> (35.9306, 211.9509) centre (35.9306, 191.9509) ccw projected
  line L2 (11.2074, 211.9509) -> (35.9306, 211.9509) projected
  arc A8 (11.2074, 211.9509) -> (0.2192, 208.662) centre (11.2074, 191.9509) ccw projected
  arc A9 (0.2192, 208.662) -> (-6.6532, 203.0317) centre (23.569, 173.1509) ccw projected
  arc A10 (-6.6532, 203.0317) -> (-12.431, 188.9702) centre (7.569, 188.9702) ccw projected
  line L3 (-12.431, 157.3316) -> (-12.431, 188.9702) projected
  arc A11 (-12.431, 157.3316) -> (-6.6532, 143.27) centre (7.569, 157.3316) ccw projected
  arc A12 (-6.6532, 143.27) -> (0.2192, 137.6398) centre (23.569, 173.1509) ccw projected
  circle A13 centre (-12.181, 208.9009) radius 1.2 projected
  circle A14 centre (59.319, 208.9009) radius 1.2 projected
  circle A15 centre (59.319, 137.4009) radius 1.2 projected
  arc A16 (-6.6532, 60.27) -> (0.2192, 54.6398) centre (23.569, 90.1509) ccw projected
  arc A17 (-12.431, 74.3316) -> (-6.6532, 60.27) centre (7.569, 74.3316) ccw projected
  line L4 (-12.431, 74.3316) -> (-12.431, 105.9702) projected
  arc A18 (-6.6532, 120.0317) -> (-12.431, 105.9702) centre (7.569, 105.9702) ccw projected
  arc A19 (0.2192, 125.662) -> (-6.6532, 120.0317) centre (23.569, 90.1509) ccw projected
  arc A20 (11.2074, 128.9509) -> (0.2192, 125.662) centre (11.2074, 108.9509) ccw projected
  line L5 (11.2074, 128.9509) -> (35.9306, 128.9509) projected
  arc A21 (46.9188, 125.662) -> (35.9306, 128.9509) centre (35.9306, 108.9509) ccw projected
  arc A22 (53.7912, 120.0317) -> (46.9188, 125.662) centre (23.569, 90.1509) ccw projected
  arc A23 (59.569, 105.9702) -> (53.7912, 120.0317) centre (39.569, 105.9702) ccw projected
  line L6 (59.569, 105.9702) -> (59.569, 74.3316) projected
  arc A24 (53.7912, 60.27) -> (59.569, 74.3316) centre (39.569, 74.3316) ccw projected
  arc A25 (46.9188, 54.6398) -> (53.7912, 60.27) centre (23.569, 90.1509) ccw projected
  arc A26 (35.9306, 51.3509) -> (46.9188, 54.6398) centre (35.9306, 71.3509) ccw projected
  line L7 (35.9306, 51.3509) -> (11.2074, 51.3509) projected
  arc A27 (0.2192, 54.6398) -> (11.2074, 51.3509) centre (11.2074, 71.3509) ccw projected
  circle A28 centre (-12.181, 54.4009) radius 1.2 projected
  circle A29 centre (59.319, 54.4009) radius 1.2 projected
  circle A30 centre (59.319, 125.9009) radius 1.2 projected
  circle A31 centre (-12.181, 125.9009) radius 1.2 projected
  point P0 (0, 0)
extrude "Extrusion12" add sketch "Sketch11" against normal up to surface (3 mm away)